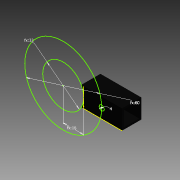
# Autodesk Inventor part: KétvégenMartSzelvény
Saved by Autodesk Inventor 2015 SP1 (Build 190203100, 203)
## iProperties
Created: 2014-08-08
Part Number: KétvégenMartSzelvény
Material: Acetal Resin, Black
Document SubType Name: Modeling
Designer: laca
Density: 1.425 g/cm^3
Appearance: Smooth - Black
Mass: 3.52497 g
Surface Area: 35.0644 cm^2
Volume: 2.47366 cm^3
Author: laca
Autodesk Inventor part; units mm, degrees
ref_plane "YZ Plane" through (0, 0, 0) normal (1, 0, 0) x (0, 1, 0)
ref_plane "XZ Plane" through (0, 0, 0) normal (0, 1, 0) x (-1, 0, 0)
ref_plane "XY Plane" through (0, 0, 0) normal (0, 0, 1) x (1, 0, 0)
sketch "Sketch1" plane through (0, 0, 0) normal (1, 0, 0) x (0, 1, 0)
  line L0 (0, 0) -> (12, 0)
  line L1 (12, 0) -> (12, 12)
  line L2 (12, 12) -> (0, 12)
  line L3 (0, 12) -> (0, 0)
  line L4 (-1.5, 13.5) -> (13.5, 13.5)
  line L5 (13.5, 13.5) -> (13.5, -1.5)
  line L6 (13.5, -1.5) -> (-1.5, -1.5)
  line L7 (-1.5, -1.5) -> (-1.5, 13.5)
  dimension "d0" = 1.5
  dimension "d1" = 12
  dimension "d2" = 12
  constraints: 16 end point, 4 parallel, 2 perpendicular, 1 horizontal, 3 other
  measures "d0" distance between parallel lines of L4 L2
  measures "d1" distance of L2.end L0.start
  measures "d2" distance of L0.start L0.end
extrude "Extrusion1" add sketch "Sketch1" along normal blind 30 and the other way blind 15
sketch "Sketch2" plane through (0, -1.5, 13.5) normal (0, 0, 1) x (1, 0, 0)
  line L0 (0, 0) -> (0, 15) projected
  line L1 (0, 0) -> (30, 0) projected
  circle A0 centre (-16, 7.5) radius 16
  circle A1 centre (-16, 7.5) radius 30
  circle A2 centre (14, 7.5) radius 2
  point P0 (0, 1.5)
  dimension "d17" = 60
  dimension "d8" = 32
  dimension "d9" = 16
  dimension "d18" = 4
  constraints: 2 centre point, 1 coincident, 1 horizontal alignment, 2 other
  measures "d8" diameter of A0
  measures "d9" distance from line of L0 A0.centre
  measures "d18" diameter of A2
sketch "Sketch4" plane through (0, 0, 0) normal (-1, 0, 0) x (0, 0, 1)
  line L0 (0, 0) -> (12, 0)
  line L1 (12, 0) -> (12, 12)
  line L2 (12, 12) -> (0, 12)
  line L3 (0, 12) -> (0, 0)
  line L4 (-1.5, -1.5) -> (13.5, -1.5)
  line L5 (13.5, -1.5) -> (13.5, 13.5)
  line L6 (13.5, 13.5) -> (-1.5, 13.5)
  line L7 (-1.5, 13.5) -> (-1.5, -1.5)
  constraints: 16 end point, 4 parallel, 2 horizontal, 2 perpendicular
extrude "Extrusion2" add sketch "Sketch4" along normal blind 10
extrude "Extrusion3" cut sketch "Sketch2" against normal through all contours A0
extrude "Extrusion4" cut sketch "Sketch2" along normal through all both and the other way through all contours A2 A1 | A1 A2 picked at (14.5954, 6.9828) picked at (13.3724, 7.0462)
equation "\"d0\" = ZártSzelvényFalVastagság"
equation "\"d1\" = ZártSzelvényBelsőÁtmérő"
equation "\"d2\" = ZártSzelvényBelsőÁtmérő"
equation "\"d17\" = 2 * PorvedoRogzitesJatekSugara"
equation "\"d8\" = CsapágyHázKülsőÁtmérő"
equation "\"d9\" = 0.5 * CsapágyHázKülsőÁtmérő"
equation "\"ZártSzelvényFalVastagság\" = 1.5"
equation "\"ZártSzelvényBelsőÁtmérő\" = 12"
equation "\"CsapágyHázKülsőÁtmérő\" = 32"
equation "\"ZártSzelvényKülsőÁtmérő\" = 15"
equation "\"CsapágyBelsőÁtmérő\" = 12"
equation "\"CsapágyKülsőÁtmérő\" = 28"
equation "\"CsapágyHázBelsőÁtmérő\" = 26"
equation "\"CsapágyHázHoszza\" = 45"
equation "\"CsapágySzélesége\" = 8"
equation "\"PorvedoRogzitesJatekSugara\" = 30"
body "Solid1"
